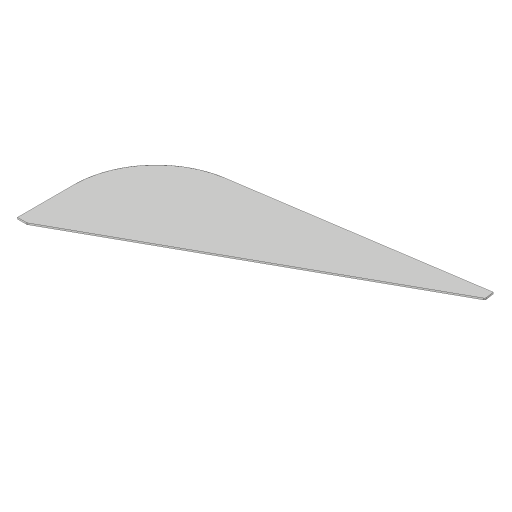
# Autodesk Inventor part: Keil
Saved by Autodesk Inventor 2023.2 (Build 272271000, 271)
## iProperties
Created: 2023-02-05
Part Number: Keil
Material: Generisch
Document SubType Name: Modeling
Designer: Raoul Messerli
Density: 1 g/cm^3
Appearance: Vorgabe
Author: Raoul Messerli
Autodesk Inventor part; units mm, degrees
ref_plane "YZ Plane" through (0, 0, 0) normal (1, 0, 0) x (0, 1, 0)
ref_plane "XZ Plane" through (0, 0, 0) normal (0, 1, 0) x (-1, 0, 0)
ref_plane "XY Plane" through (0, 0, 0) normal (0, 0, 1) x (1, 0, 0)
sketch "Skizze1" plane through (0, 0, 0) normal (0, 0, 1) x (1, 0, 0)
  line L0 (0, 0) -> (0, 180)
  arc A0 (222.6888, 438.991) -> (0, 180) centre (261.95, 180) ccw
  line L1 (222.6888, 438.991) -> (964.2169, 551.4014)
  line L2 (0, 0) -> (30, 0)
  line L3 (964.2169, 551.4014) -> (968.7133, 521.7403)
  line L4 (968.7133, 521.7403) -> (30, 0)
  dimension "d0" = 98.62
  dimension "d2" = 30
  dimension "d5" = 261.95
  dimension "d6" = 180
  dimension "d8" = 750
  dimension "d11" = 30
  constraints: 10 end point, 2 point on circle, 2 tangent, 1 centre point, 1 equal length, 1 horizontal, 1 perpendicular, 1 vertical
  measures "d0" angle of L1 L0
  measures "d2" distance of L0.start L2.end
  measures "d5" radius of A0
  measures "d6" distance of L0.start L0.end
  measures "d8" distance of L1.start L1.end
  measures "d11" distance of L1.end L3.end
extrude "Extrusion1" add sketch "Skizze1" along normal mid plane 5
fillet "Rundung1" radius 5 2 edges at (968.7133, 521.7403, 0) (30, 0, 0)
